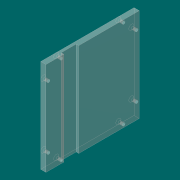
# Autodesk Inventor part: sides
Saved by Autodesk Inventor 2016 (Build 200138000, 138)
## iProperties
Created: 2015-10-13
Part Number: sides
Material: PC/ABS Plastic
Document SubType Name: Modeling
Designer: Sawaiz
Density: 0.357273 g/cm^3
Appearance: Polycarbonate - Clear
Author: Sawaiz
Autodesk Inventor part; units mm, degrees
ref_plane "YZ Plane" through (0, 0, 0) normal (1, 0, 0) x (0, 1, 0)
ref_plane "XZ Plane" through (0, 0, 0) normal (0, 1, 0) x (-1, 0, 0)
ref_plane "XY Plane" through (0, 0, 0) normal (0, 0, 1) x (1, 0, 0)
sketch "Sketch1" plane through (0, 0, 0) normal (0, 1, 0) x (-1, 0, 0)
  line L0 (-56.35, 56.35) -> (56.35, 56.35)
  line L1 (56.35, 56.35) -> (56.35, -56.35)
  line L2 (56.35, -56.35) -> (-56.35, -56.35)
  line L3 (-56.35, -56.35) -> (-56.35, 56.35)
  line L4 (-56.35, 56.35) -> (56.35, -56.35) construction
  line L5 (56.35, 56.35) -> (-56.35, -56.35) construction
  point P0 (0, 0)
  dimension "d0" = 112.7
  dimension "d1" = 112.7
  constraints: 12 end point, 2 midpoint, 2 parallel, 1 horizontal, 1 perpendicular
  measures "d0" distance of L1.end L2.end
  measures "d1" distance of L0.end L1.end
extrude "Extrusion1" add sketch "Sketch1" along normal blind 6.35
sketch "Sketch2" plane through (0, 6.35, 0) normal (0, 1, 0) x (1, 0, 0)
  line L0 (-56.35, -56.35) -> (56.35, -56.35) projected
  line L1 (56.35, -56.35) -> (56.35, 56.35) projected
  line L2 (56.35, 56.35) -> (-56.35, 56.35) projected
  line L3 (-56.35, 56.35) -> (-56.35, -56.35) projected
  line L4 (-56.35, -56.35) -> (56.35, -56.35) projected
  line L5 (34.726, 56.35) -> (16.726, 56.35)
  line L6 (16.726, 56.35) -> (16.726, -56.35)
  line L7 (16.726, -56.35) -> (34.726, -56.35)
  line L8 (34.726, -56.35) -> (34.726, 56.35)
  line L9 (34.726, 56.35) -> (16.726, -56.35) construction
  line L10 (16.726, 56.35) -> (34.726, -56.35) construction
  point P0 (0, 0)
  point P1 (25.726, 0)
  dimension "d4" = 18
  dimension "d5" = 21.624
  constraints: 12 end point, 2 midpoint, 2 parallel, 1 collinear, 1 horizontal, 1 perpendicular, 1 point on line
  measures "d4" distance between parallel lines of L6 L8
  measures "d5" distance between parallel lines of L1 L8
extrude "Extrusion2" cut sketch "Sketch2" against normal blind 3.175 contours L6 L2 L8 L0
sketch "Sketch3" plane through (0, 0, 0) normal (0, -1, 0) x (1, 0, 0)
  line L0 (56.35, 56.35) -> (-56.35, 56.35) projected
  line L1 (-56.35, 56.35) -> (-56.35, -56.35) projected
  line L2 (-56.35, -56.35) -> (56.35, -56.35) projected
  line L3 (56.35, -56.35) -> (56.35, 56.35) projected
  line L4 (-53.175, 56.35) -> (-53.175, -56.35)
  point P0 (0, 0)
  point P1 (-53.175, 37.5)
  point P2 (-53.175, 12.5)
  point P3 (-53.175, -12.5)
  point P4 (-53.175, -37.5)
  dimension "d8" = 3.175
  dimension "d9" = 12.5
  dimension "d10" = 12.5
  dimension "d11" = 25
  dimension "d12" = 25
  constraints: 6 point on line, 2 end point, 1 perpendicular
  measures "d8" distance between parallel lines of L1 L4
  measures "d9" vertical distance of point (-53.175, 12.5) point (0, 0)
  measures "d10" vertical distance of point (0, 0) point (-53.175, -12.5)
  measures "d11" distance of point (-53.175, 12.5) point (-53.175, 37.5)
  measures "d12" distance of point (-53.175, -12.5) point (-53.175, -37.5)
hole "Hole1" at (-53.175, 0, 37.5) at (-53.175, 0, -37.5) direction (0, 1, 0) diameter 3.4 end through all countersink diameter 6.3 countersink angle 90 clearance for "Flat Head Machine Screw" size "M3" standard "Ansi Metric M Profile"
mirror "Mirror1" about plane through (0, 0, 0) normal (1, 0, 0) of "Hole1"
sketch "Sketch4" plane through (0, 0, 0) normal (0, -1, 0) x (1, 0, 0)
  circle A0 centre (53.175, -37.5) radius 3.15 projected
  circle A1 centre (53.175, 37.5) radius 3.15 projected
  circle A2 centre (-53.175, 37.5) radius 3.15 projected
  circle A3 centre (-53.175, -37.5) radius 3.15 projected
  line L0 (56.35, 56.35) -> (-56.35, 56.35) projected
  line L1 (-56.35, 56.35) -> (-56.35, -56.35) projected
  line L2 (-56.35, -56.35) -> (56.35, -56.35) projected
  line L3 (56.35, -56.35) -> (56.35, 56.35) projected
  line L4 (-56.35, 53.175) -> (56.35, 53.175)
  line L5 (56.35, -56.35) -> (56.35, 56.35) projected
  point P0 (0, 0)
  point P1 (-37.5, 53.175)
  point P2 (-12.5, 53.175)
  point P3 (12.5, 53.175)
  point P4 (37.5, 53.175)
  dimension "d20" = 3.175
  dimension "d21" = 12.5
  dimension "d22" = 12.5
  dimension "d23" = 25
  dimension "d24" = 25
  constraints: 6 point on line, 2 end point, 1 horizontal
  measures "d20" distance between parallel lines of L0 L4
  measures "d21" horizontal distance of point (0, 0) point (-12.5, 53.175)
  measures "d22" horizontal distance of point (0, 0) point (12.5, 53.175)
  measures "d23" distance of point (12.5, 53.175) point (37.5, 53.175)
  measures "d24" distance of point (-37.5, 53.175) point (-12.5, 53.175)
hole "Hole2" at (-37.5, 0, 53.175) at (37.5, 0, 53.175) direction (0, 1, 0) diameter 3.4 end through all countersink diameter 6.3 countersink angle 90 clearance for "Flat Head Machine Screw" size "M3" standard "Ansi Metric M Profile"
mirror "Mirror2" about plane through (0, 0, 0) normal (0, 0, 1) of "Hole2"
equation "\"d0\" = depth + 2 * acrylicThickness"
equation "\"d1\" = depth + 2 * acrylicThickness"
equation "\"d2\" = acrylicThickness"
equation "\"d4\" = 6 * mirrorThickness"
equation "\"d5\" = centerThickness + aerogelThickness + fresnelThickness"
equation "\"d6\" = 0.5 * acrylicThickness"
equation "\"d8\" = 0.5 * acrylicThickness"
equation "\"d9\" = 0.125 * height"
equation "\"d10\" = 0.125 * height"
equation "\"d11\" = 0.25 * height"
equation "\"d12\" = 0.25 * height"
equation "\"d20\" = 0.5 * acrylicThickness"
equation "\"d21\" = 0.125 * depth"
equation "\"d22\" = 0.125 * depth"
equation "\"d23\" = 0.25 * depth"
equation "\"d24\" = 0.25 * depth"
equation "\"acrylicThickness\" = 6.35"
equation "\"mirrorThickness\" = 3"
equation "\"aerogelThickness\" = 20"
equation "\"mirrorAngle\" = 17deg"
equation "\"detectorWidth\" = 52"
equation "\"detectorHeight\" = 52"
equation "\"fresnelThickness\" = 0.1"
equation "\"focalLength\" = 76.2"
equation "\"ior\" = 1.49"
equation "\"centerThickness\" = 1.524"
equation "\"fresnelAngle\" = 90deg"
equation "\"fresnelEffectiveDiameter\" = 76.2"
equation "\"depth\" = 100"
equation "\"height\" = 100"
body "Solid1"
